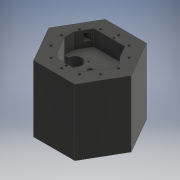
# Autodesk Inventor part: AC02
Saved by Autodesk Inventor 2017 SP1 (Build 210196100, 196)
## iProperties
Created: 2019-08-28
Part Number: AC02
Material: ABS Plastic
Document SubType Name: Modeling
Designer: Dell
Density: 1.06 g/cm^3
Appearance: Smooth - Black
Author: Dell
Autodesk Inventor part; units mm, degrees
ref_plane "YZ Plane" through (0, 0, 0) normal (1, 0, 0) x (0, 1, 0)
ref_plane "XZ Plane" through (0, 0, 0) normal (0, 1, 0) x (-1, 0, 0)
ref_plane "XY Plane" through (0, 0, 0) normal (0, 0, 1) x (1, 0, 0)
sketch "Sketch1" plane through (0, 0, 0) normal (0, 0, 1) x (1, 0, 0)
  circle A0 centre (0, 0) radius 4.7625
  circle A1 centre (0, 0) radius 67.5
  dimension "d0" = 9.525
  dimension "d1" = 135
  constraints: 2 centre point, 2 coincident
  measures "d0" diameter of A0
  measures "d1" diameter of A1
extrude "Extrusion1" add sketch "Sketch1" along normal blind 10
sketch "Sketch3" plane through (0, 0, 10) normal (0, 0, 1) x (1, 0, 0)
  circle A0 centre (28, 0) radius 11
  circle A1 centre (-28, 0) radius 11
  circle A2 centre (-28, 0) radius 5.5
  point P0 (0, 0)
  dimension "d12" = 22
  dimension "d13" = 28
  dimension "d16" = 360
  dimension "d18" = 11
  constraints: 3 centre point, 1 coincident, 1 horizontal alignment, 5 other
  measures "d12" diameter of A0
  measures "d13" distance of A0.centre point (0, 0)
  measures "d18" diameter of A2
extrude "Extrusion3" cut sketch "Sketch3" against normal through all contours A0 | A2
sketch "Sketch4" plane through (0, 0, 10) normal (0, 0, 1) x (1, 0, 0)
  circle A0 centre (0, 0) radius 67.5 projected
  circle A1 centre (0, 0) radius 62.5
  dimension "d21" = 5
  constraints: 1 centre point
  measures "d21" radial gap between concentric circles of A0 A1
extrude "Extrusion4" add sketch "Sketch4" along normal blind 105
sketch "Sketch5" plane through (0, 0, 0) normal (0, 0, -1) x (-1, 0, 0)
  circle A0 centre (-54, 0) radius 2
  circle A1 centre (-46.7654, -27) radius 2
  circle A2 centre (-27, -46.7654) radius 2
  circle A3 centre (0, -54) radius 2
  circle A4 centre (27, -46.7654) radius 2
  circle A5 centre (46.7654, -27) radius 2
  circle A6 centre (54, 0) radius 2
  circle A7 centre (46.7654, 27) radius 2
  circle A8 centre (27, 46.7654) radius 2
  circle A9 centre (0, 54) radius 2
  circle A10 centre (-27, 46.7654) radius 2
  circle A11 centre (-46.7654, 27) radius 2
  point P0 (0, 0)
  dimension "d24" = 4
  dimension "d25" = 54
  dimension "d28" = 360
  constraints: 12 centre point, 1 horizontal alignment, 25 other
  measures "d24" diameter of A0
  measures "d25" distance of point (0, 0) A0.centre
extrude "Extrusion5" cut sketch "Sketch5" against normal through all
sketch "Sketch6" plane through (0, 0, 0) normal (0, 0, -1) x (-1, 0, 0)
  circle A0 centre (-28, 0) radius 11 projected
  circle A1 centre (-19, -9) radius 2
  line L0 (-28, 0) -> (0, 0) construction
  line L1 (-19, -9) -> (-28, 0) construction
  circle A2 centre (-19, 9) radius 2
  circle A3 centre (-37, 9) radius 2
  circle A4 centre (-37, -9) radius 2
  dimension "d32" = 12.7279
  dimension "d33" = 45
  dimension "d34" = 4
  dimension "d37" = 360
  constraints: 4 centre point, 4 end point, 1 horizontal, 9 other
  measures "d32" distance of L1.start L0.start
  measures "d33" angle of L0 L1
  measures "d34" diameter of A1
extrude "Extrusion6" cut sketch "Sketch6" against normal through all contours A2 A0 | A0 A2 | A1 A0 | A0 A1 | A3 A0 | A0 A3 | A4 A0 | A0 A4
sketch "Sketch7" plane through (0, 0, 0) normal (0, 0, -1) x (-1, 0, 0)
  arc A0 (-36.4114, -7.0886) -> (-35.0886, -8.4114) centre (-37, -9) ccw projected
  arc A1 (-35.0886, -8.4114) -> (-20.9114, -8.4114) centre (-28, 0) ccw projected
  circle A2 centre (-37, -9) radius 4.5
  circle A3 centre (-19, -9) radius 4.5
  circle A4 centre (-19, 9) radius 4.5
  circle A5 centre (-37, 9) radius 4.5
  point P0 (0, 0)
  dimension "d41" = 9
  dimension "d44" = 360
  constraints: 4 centre point, 1 coincident, 9 other
  measures "d41" diameter of A2
extrude "Extrusion7" cut sketch "Sketch7" against normal blind 4
sketch "Sketch9" plane through (0, 0, 0) normal (0, 0, -1) x (-1, 0, 0)
  line L0 (77.9423, 0) -> (38.9711, -67.5)
  line L1 (38.9711, -67.5) -> (-38.9711, -67.5)
  line L2 (-38.9711, -67.5) -> (-77.9423, 0)
  line L3 (-77.9423, 0) -> (-38.9711, 67.5)
  line L4 (-38.9711, 67.5) -> (38.9711, 67.5)
  line L5 (38.9711, 67.5) -> (77.9423, 0)
  circle A0 centre (0, 0) radius 67.5 projected
  constraints: 12 end point, 1 coincident, 1 horizontal alignment, 1 tangent, 13 other
extrude "Extrusion9" add sketch "Sketch9" against normal blind 115 contours L0 A0 L5 | L0 L1 A0 | A0 L4 L5 | L1 L2 A0 | A0 L3 L4 | L2 L3 A0
sketch "Sketch10" plane through (0, 0, 0) normal (0, 0, -1) x (-1, 0, 0)
  circle A0 centre (28, 0) radius 5.5 projected
  circle A1 centre (28, -8.5) radius 1.5
  circle A2 centre (28, 8.5) radius 1.5
  point P0 (0, 0)
  dimension "d53" = 3
  dimension "d54" = 8.5
  dimension "d57" = 360
  constraints: 2 centre point, 1 vertical alignment, 5 other
  measures "d53" diameter of A1
  measures "d54" distance of A0.centre A1.centre
extrude "Extrusion10" cut sketch "Sketch10" against normal through all contours A1 | A2
sketch "Sketch11" plane through (0, 0, 0) normal (0, 0, -1) x (-1, 0, 0)
  circle A0 centre (28, -8.5) radius 1.5 projected
  circle A1 centre (28, 0) radius 5.5 construction
  circle A2 centre (28, -8.5) radius 4
  circle A3 centre (28, 8.5) radius 4
  point P0 (0, 0)
  dimension "d61" = 8
  dimension "d64" = 360
  constraints: 2 centre point, 1 coincident, 5 other
  measures "d61" diameter of A2
extrude "Extrusion11" cut sketch "Sketch11" against normal blind 8 contours A0 | A2 | A3
sketch "Sketch12" plane through (0, 0, 0) normal (0, 0, -1) x (-1, 0, 0)
  arc A0 (25.912, 5.0882) -> (25.912, -5.0882) centre (28, 0) ccw projected
  circle A1 centre (28, 0) radius 11
  point P0 (0, 0)
  dimension "d68" = 22
  constraints: 1 centre point, 1 coincident
  measures "d68" diameter of A1
extrude "Extrusion12" cut sketch "Sketch12" against normal blind 5
sketch "Sketch13" plane through (0, 0, 115) normal (0, 0, 1) x (1, 0, 0)
  circle A0 centre (0, 0) radius 62.5 projected
  line L0 (-38.9711, -67.5) -> (38.9711, -67.5) projected
  line L1 (38.9711, -67.5) -> (77.9423, 0) projected
  line L2 (77.9423, 0) -> (38.9711, 67.5) projected
  line L3 (38.9711, 67.5) -> (-38.9711, 67.5) projected
  line L4 (-38.9711, 67.5) -> (-77.9423, 0) projected
  line L5 (-77.9423, 0) -> (-38.9711, -67.5) projected
extrude "Extrusion13" add sketch "Sketch13" along normal blind 10
sketch "Sketch14" plane through (0, 0, 10) normal (0, 0, 1) x (1, 0, 0)
  circle A0 centre (0, 0) radius 47.5 construction
  arc A1 (35.0886, 8.4114) -> (20.9114, 8.4114) centre (28, 0) ccw projected
  circle A2 centre (28, 0) radius 21
  circle A3 centre (-28, 0) radius 5.5 projected
  circle A4 centre (-28, 0) radius 12.5
  circle A5 centre (0, 0) radius 4.7625 projected
  circle A6 centre (0, 0) radius 62.5 projected
  circle A7 centre (-28, -8.5) radius 1.5 projected
  circle A8 centre (-28, 8.5) radius 1.5 projected
  arc A9 (35.0886, -8.4114) -> (36.4114, -7.0886) centre (37, -9) ccw projected
  arc A10 (20.9114, -8.4114) -> (35.0886, -8.4114) centre (28, 0) ccw projected
  arc A11 (19.5886, -7.0886) -> (20.9114, -8.4114) centre (19, -9) ccw projected
  arc A12 (19.5886, 7.0886) -> (19.5886, -7.0886) centre (28, 0) ccw projected
  arc A13 (20.9114, 8.4114) -> (19.5886, 7.0886) centre (19, 9) ccw projected
  arc A14 (35.0886, 8.4114) -> (20.9114, 8.4114) centre (28, 0) ccw projected
  arc A15 (36.4114, 7.0886) -> (35.0886, 8.4114) centre (37, 9) ccw projected
  arc A16 (36.4114, -7.0886) -> (36.4114, 7.0886) centre (28, 0) ccw projected
  circle A17 centre (27, 46.7654) radius 2 projected
  circle A18 centre (-27, 46.7654) radius 2 projected
  circle A19 centre (-54, 0) radius 2 projected
  circle A20 centre (-27, -46.7654) radius 2 projected
  circle A21 centre (27, -46.7654) radius 2 projected
  circle A22 centre (54, 0) radius 2 projected
  circle A23 centre (46.7654, -27) radius 2 projected
  circle A24 centre (0, -54) radius 2 projected
  circle A25 centre (-46.7654, -27) radius 2 projected
  circle A26 centre (-46.7654, 27) radius 2 projected
  circle A27 centre (0, 54) radius 2 projected
  circle A28 centre (46.7654, 27) radius 2 projected
  circle A29 centre (0, 0) radius 62.5 projected
  circle A30 centre (-28, 0) radius 5.5 projected
  circle A31 centre (0, 0) radius 4.7625 projected
  dimension "d73" = 95
  dimension "d74" = 42
  dimension "d75" = 25
  constraints: 3 centre point, 3 coincident
  measures "d73" diameter of A0
  measures "d74" diameter of A2
  measures "d75" diameter of A4
extrude "Extrusion14" add sketch "Sketch14" along normal blind 85 contours A6
sketch "Sketch15" plane through (0, 0, 95) normal (0, 0, 1) x (1, 0, 0)
  circle A0 centre (0, 0) radius 4.7625 projected
  line L0 (48.2624, 0) -> (24.1312, -41.7965)
  line L1 (24.1312, -41.7965) -> (-24.1312, -41.7965)
  line L2 (-24.1312, -41.7965) -> (-48.2624, 0)
  line L3 (-48.2624, 0) -> (-24.1312, 41.7965)
  line L4 (-24.1312, 41.7965) -> (24.1312, 41.7965)
  line L5 (24.1312, 41.7965) -> (48.2624, 0)
  circle A1 centre (0, 0) radius 62.5 projected
  circle A2 centre (28, 0) radius 21 projected
  circle A3 centre (-28, 0) radius 12.5 projected
  circle A4 centre (0, 0) radius 4.7625 projected
  circle A5 centre (46.7654, 27) radius 2 projected
  circle A6 centre (0, 54) radius 2 projected
  circle A7 centre (-46.7654, 27) radius 2 projected
  circle A8 centre (-46.7654, -27) radius 2 projected
  circle A9 centre (0, -54) radius 2 projected
  circle A10 centre (46.7654, -27) radius 2 projected
  circle A11 centre (54, 0) radius 2 projected
  circle A12 centre (27, -46.7654) radius 2 projected
  circle A13 centre (-27, -46.7654) radius 2 projected
  circle A14 centre (-54, 0) radius 2 projected
  circle A15 centre (-27, 46.7654) radius 2 projected
  circle A16 centre (27, 46.7654) radius 2 projected
  circle A17 centre (0, 0) radius 62.5 projected
  dimension "d78" = 83.5929
  constraints: 12 end point, 1 coincident, 1 horizontal alignment, 13 other
  measures "d78" distance between parallel lines of L1 L4
extrude "Extrusion15" add sketch "Sketch15" along normal blind 30 contours A1
sketch "Sketch16" plane through (0, 0, 95) normal (0, 0, 1) x (1, 0, 0)
  circle A0 centre (0, 45) radius 2
  circle A1 centre (-45, 0) radius 2
  circle A2 centre (0, -45) radius 2
  circle A3 centre (45, 0) radius 2
  point P0 (0, 0)
  dimension "d81" = 4
  dimension "d83" = 45
  dimension "d89" = 360
  constraints: 4 centre point, 1 vertical alignment, 9 other
  measures "d81" diameter of A0
  measures "d83" distance of point (0, 0) A0.centre
extrude "Extrusion16" cut sketch "Sketch16" along normal through all both and the other way through all contours A0 | A2
sketch "Sketch17" plane through (0, 0, 95) normal (0, 0, 1) x (1, 0, 0)
  line L0 (24.1312, -41.7965) -> (-24.1312, -41.7965) projected
  line L1 (10, -41.7965) -> (10, -21.7965)
  line L2 (10, -21.7965) -> (-12.5842, -21.7965)
  line L3 (-12.5842, -21.7965) -> (-25.1684, 0)
  line L4 (-25.1684, 0) -> (-12.5842, 21.7965)
  line L5 (-12.5842, 21.7965) -> (10, 21.7965)
  line L6 (10, 21.7965) -> (10, 41.7965)
  line L7 (-24.1312, 41.7965) -> (24.1312, 41.7965) projected
  line L8 (-24.1312, 41.7965) -> (10, 41.7965)
  line L9 (10, -41.7965) -> (-24.1312, -41.7965)
  line L10 (-24.1312, -41.7965) -> (-48.2624, 0) projected
  line L11 (-48.2624, 0) -> (-24.1312, 41.7965) projected
  line L12 (-25.1684, 0) -> (-48.2624, 0)
  point P0 (0, 0)
  dimension "d91" = 20
  dimension "d92" = 20
  dimension "d94" = 20
  dimension "d95" = 10
  constraints: 18 end point, 4 point on line, 3 parallel, 2 collinear, 1 horizontal, 1 horizontal alignment, 1 perpendicular, 1 vertical
  measures "d91" distance between parallel lines of L0 L2
  measures "d92" distance between parallel lines of L10 L3
  measures "d94" distance of L5.end L6.end
  measures "d95" distance from line of point (0, 0) L6
extrude "Extrusion18" cut sketch "Sketch17" against normal blind 20 contours L0 L10 L12 L3 L2 L1
sketch "Sketch19" plane through (0, 0, 95) normal (0, 0, 1) x (1, 0, 0)
  circle A0 centre (-15.5, 12.5) radius 1.5
  point P0 (0, 0)
  dimension "d100" = 3
  dimension "d101" = 12.5
  dimension "d102" = 15.5
  constraints: 1 centre point
  measures "d100" diameter of A0
  measures "d101" vertical distance of point (0, 0) A0.centre
  measures "d102" horizontal distance of A0.centre point (0, 0)
extrude "Extrusion19" cut sketch "Sketch19" against normal through all
sketch "Sketch20" plane through (0, 0, 95) normal (0, 0, 1) x (1, 0, 0)
  line L0 (-24.1312, 41.7965) -> (-48.2624, 0) projected
  line L1 (-38.9711, 67.5) -> (-77.9423, 0) projected
  line L2 (-25.8632, 38.7965) -> (-60.7393, 38.7965)
  line L3 (-60.7393, 38.7965) -> (-60.7393, 29.7965)
  line L4 (-60.7393, 29.7965) -> (-25.8632, 29.7965)
  line L5 (-25.8632, 29.7965) -> (-25.8632, 38.7965)
  line L6 (-24.1312, 41.7965) -> (24.1312, 41.7965) projected
  point P0 (0, 0)
  dimension "d105" = 3
  dimension "d111" = 9
  constraints: 8 end point, 2 parallel, 2 point on line, 1 horizontal, 1 perpendicular
  measures "d105" distance between parallel lines of L6 L2
  measures "d111" distance of L4.end L2.start
extrude "Extrusion20" cut sketch "Sketch20" along normal blind 25
sketch "Sketch21" plane through (0, 0, 95) normal (0, 0, 1) x (1, 0, 0)
  circle A0 centre (0, 0) radius 4.7625 projected
  line L0 (-31.0594, 29.7965) -> (-48.2624, 0) projected
  line L1 (-48.2624, 0) -> (-40.5, 0) projected
  arc A1 (-19.7477, -9.3888) -> (-40.5, 0) centre (-28, 0) ccw projected
  line L2 (-19.7477, -9.3888) -> (-12.5842, -21.7965) projected
  line L3 (-12.5842, -21.7965) -> (10, -21.7965) projected
  line L4 (10, -21.7965) -> (10, -41.7965) projected
  line L5 (10, -41.7965) -> (24.1312, -41.7965) projected
  line L6 (24.1312, -41.7965) -> (37.4289, -18.7642) projected
  arc A2 (37.4289, 18.7642) -> (37.4289, -18.7642) centre (28, 0) ccw projected
  line L7 (37.4289, 18.7642) -> (24.1312, 41.7965) projected
  line L8 (24.1312, 41.7965) -> (-24.1312, 41.7965) projected
  line L9 (-24.1312, 41.7965) -> (-25.8632, 38.7965) projected
  line L10 (-25.8632, 38.7965) -> (-55.5431, 38.7965) projected
  line L11 (-60.7393, 29.7965) -> (-55.5431, 38.7965) projected
  line L12 (-60.7393, 29.7965) -> (-31.0594, 29.7965) projected
  circle A3 centre (-15.5, 12.5) radius 1.5 projected
  line L13 (-25.8632, 38.7965) -> (-31.0594, 29.7965)
  constraints: 2 end point, 1 collinear
extrude "Extrusion21" add sketch "Sketch21" along normal blind 11 contours L12 L11 L10 L13
sketch "Sketch22" plane through (0, 0, 95) normal (0, 0, 1) x (1, 0, 0)
  line L0 (-48.2624, 0) -> (-24.1312, 41.7965) projected
  line L1 (-48.2624, 18) -> (-34.5235, 41.7965)
  line L2 (-34.5235, 41.7965) -> (-24.1312, 41.7965)
  line L3 (-48.2624, 18) -> (-48.2624, 0)
  point P0 (0, 0)
  dimension "d112" = 9
  constraints: 6 end point, 1 horizontal, 1 parallel, 1 vertical
  measures "d112" distance between parallel lines of L0 L1
extrude "Extrusion22" cut sketch "Sketch22" along normal through all
sketch "Sketch24" plane through (0, 0, 0) normal (0, 0, -1) x (-1, 0, 0)
  circle A0 centre (0, 0) radius 4.7625 projected
  circle A1 centre (0, -30) radius 5.5
  dimension "d119" = 11
  dimension "d120" = 30
  constraints: 1 centre point, 1 vertical alignment
  measures "d119" diameter of A1
  measures "d120" distance of point (0, 0) A1.centre
extrude "Extrusion24" cut sketch "Sketch24" against normal through all contours A1
sketch "Sketch25" plane through (-28, 0, 10) normal (0, 0, 1) x (1, 0, 0)
  circle A0 centre (28, -30) radius 5.5 projected
  circle A1 centre (28, -30) radius 12.5
  point P0 (28, 0)
  dimension "d123" = 25
  constraints: 1 centre point, 1 coincident
  measures "d123" diameter of A1
extrude "Extrusion25" cut sketch "Sketch25" along normal through all
sketch "Sketch26" plane through (0, -30, 10) normal (0, 0, 1) x (1, 0, 0)
  circle A0 centre (0, -8.5) radius 1.5
  circle A1 centre (0, 0) radius 5.5 construction
  circle A2 centre (0, 0) radius 12.5 construction
  circle A3 centre (0, 8.5) radius 1.5
  point P0 (0, 30)
  dimension "d126" = 3
  dimension "d127" = 8.5
  dimension "d130" = 360
  constraints: 2 centre point, 1 vertical alignment, 5 other
  measures "d126" diameter of A0
  measures "d127" distance of A1.centre A0.centre
extrude "Extrusion26" cut sketch "Sketch26" against normal through all
sketch "Sketch27" plane through (0, 0, 8) normal (0, 0, -1) x (-1, 0, 0)
  circle A0 centre (0, -38.5) radius 1.5 projected
  circle A1 centre (0, -21.5) radius 1.5 projected
  circle A2 centre (0, -38.5) radius 1.5 projected
  circle A3 centre (0, -38.5) radius 4
  circle A4 centre (0, -21.5) radius 4
  point P0 (0, 0)
  dimension "d134" = 8
  dimension "d135" = 8
  constraints: 2 centre point, 2 coincident
  measures "d134" diameter of A3
  measures "d135" diameter of A4
extrude "Extrusion27" cut sketch "Sketch27" along normal through all
sketch "Sketch28" plane through (0, 0, 5) normal (0, 0, -1) x (-1, 0, 0)
  arc A0 (2.088, -35.0882) -> (2.088, -24.9118) centre (0, -30) ccw projected
  circle A1 centre (0, -30) radius 11
  point P0 (0, 0)
  dimension "d138" = 22
  constraints: 1 centre point, 1 coincident
  measures "d138" diameter of A1
extrude "Extrusion28" cut sketch "Sketch28" along normal through all
sketch "Sketch29" plane through (0, 0, 0) normal (0, 0, -1) x (-1, 0, 0)
  circle A0 centre (0, 0) radius 17.5
  dimension "d141" = 35
  constraints: 1 centre point, 1 coincident
  measures "d141" diameter of A0
extrude "Extrusion29" cut sketch "Sketch29" against normal blind 6
body "Solid1"
